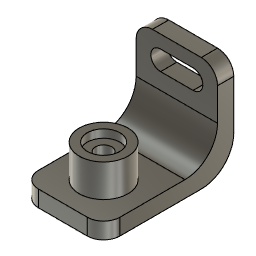
Tarea09_Ej1_jaalobuela (Autodesk Fusion 360 design; units mm, degrees)
Autodesk Fusion 360 part; units mm, degrees
sketch "Sketch1" plane through (0, 0, 0) normal (0, 0, 1) x (1, 0, 0)
  line L0 (-50, 25) -> (-41.3397, 30)
  line L1 (-50, 25) -> (-50, 35)
  line L2 (-50, 25) -> (-58.6603, 30)
  line L3 (-41.3397, 30) -> (-41.3397, 40)
  line L4 (-58.6603, 30) -> (-58.6603, 40)
  line L5 (-50, 35) -> (-41.3397, 40)
  line L6 (-50, 35) -> (-58.6603, 40)
  line L7 (-50, 45) -> (-41.3397, 40)
  line L8 (-50, 45) -> (-58.6603, 40)
sketch "Sketch2" plane through (0, 0, 0) normal (0, 0, 1) x (1, 0, 0)
  line L0 (-52.3894, 55.4322) -> (-22.3894, 55.4322)
  line L1 (-12.3894, 45.4322) -> (-12.3894, 15.4322)
  line L2 (-22.3894, 5.4322) -> (-52.3894, 5.4322)
  line L3 (-62.3894, 15.4322) -> (-62.3894, 45.4322)
  arc A0 (-12.3894, 45.4322) -> (-22.3894, 55.4322) centre (-22.3894, 45.4322) ccw
  arc A1 (-22.3894, 5.4322) -> (-12.3894, 15.4322) centre (-22.3894, 15.4322) ccw
  circle A2 through (-32.3894, 30.4322, 10) (-39.8894, 34.7623, 10) (-39.8894, 26.102, 10)
  circle A3 through (-27.3894, 30.4322, 10) (-42.3894, 39.0924, 10) (-42.3894, 21.7719, 10)
  circle A4 through (-22.3894, 30.4322, 10) (-44.8894, 43.4225, 10) (-44.8894, 17.4418, 10)
  line L4 (-37.3894, 55.4322) -> (-37.3894, 5.4322) construction
  line L5 (-62.3894, 30.4322) -> (-12.3894, 30.4322)
  line L6 (-62.3894, 15.4322) -> (-62.3894, 5.4322)
  line L7 (-62.3894, 45.4322) -> (-62.3894, 55.4322)
  line L8 (-52.3894, 55.4322) -> (-62.3894, 55.4322)
  line L9 (-52.3894, 5.4322) -> (-62.3894, 5.4322)
  point P0 (-12.3894, 55.4322)
  dimension "d8" = 50
  dimension "d9" = 50
  constraint horizontal L0
  constraint vertical L1
  constraint horizontal L2
  constraint vertical L3
  constraint coincident L7.end L0
  constraint coincident L7.end L3
  constraint coincident L6.end L3
  constraint coincident L6.end L2
  constraint coincident P0 L0
  constraint coincident P0 L1
  constraint tangent L0 A0
  constraint tangent L1 A0
  constraint tangent L1 A1
  constraint tangent L2 A1
  constraint midpoint L0 L4.start
  constraint midpoint L2 L4.end
  constraint midpoint L3 L5.start
  constraint midpoint L1 L5.end
  constraint parallel L3 L6
  constraint parallel L3 L7
  constraint perpendicular L7 L8
  constraint perpendicular L3 L9
  measures "d8" distance of L7.end P0
  measures "d9" distance of L7.end L6.end
extrude "Extrude1" add sketch "Sketch2" along normal blind 10 makes body 1
extrude "Extrude2" add sketch "Sketch2" along normal blind 15 contours A3 in plane through (0, 0, 10) normal (0, 0, 1) bodies 1
extrude "Extrude3" add sketch "Sketch2" along normal blind 20 contours A4 in plane through (0, 0, 10) normal (0, 0, 1) bodies 1
sketch "Sketch3" plane through (0, 0, 0) normal (1, 0, 0) x (0, 1, 0)
  line L0 (13, 99) -> (43, 99)
  line L1 (53, 89) -> (53, 49)
  line L2 (53, 49) -> (3, 49)
  line L3 (3, 49) -> (3, 89)
  arc A0 (13, 99) -> (3, 89) centre (13, 89) ccw
  arc A1 (53, 89) -> (43, 99) centre (43, 89) ccw
  line L4 (28, 99) -> (28, 91) construction
  line L5 (28, 91) -> (38, 91)
  line L6 (38, 79) -> (28, 79)
  line L7 (28, 91) -> (18, 91)
  line L8 (18, 79) -> (28, 79)
  arc A2 (18, 91) -> (18, 79) centre (18, 85) ccw
  arc A3 (38, 79) -> (38, 91) centre (38, 85) ccw
  point P0 (3, 99)
  point P1 (53, 99)
  dimension "d21" = 50
  dimension "d22" = 50
  dimension "d23" = 10
  dimension "d24" = 10
  dimension "d25" = 8
  dimension "d27" = 10
  constraint horizontal L0
  constraint vertical L1
  constraint horizontal L2
  constraint vertical L3
  constraint coincident P0 L0
  constraint coincident P0 L3
  constraint tangent L0 A0
  constraint tangent L3 A0
  constraint coincident P1 L0
  constraint coincident P1 L1
  constraint tangent L0 A1
  constraint tangent L1 A1
  constraint midpoint L0 L4.start
  constraint perpendicular L0 L4
  measures "d21" distance of P0 P1
  measures "d22" distance of P0 L2.end
  measures "d23" radius of A0
  measures "d24" radius of A1
  measures "d25" distance of L4.start L4.end
  measures "d27" distance of L4.end L5.end
extrude "Extrude4" add sketch "Sketch3" along normal blind 10 separate body makes body 2
move_face "OffsetFaces1" offset 20 1 faces at (-62.3894, 22.0988, 3.3333) on bodies 1
extrude "Extrude5" add 1 faces at (3.3333, 36.3333, 49) along direction (0, 0, -1) blind 10 on bodies 2 bodies 2
move_body "Move1" bodies 2 to x (1, 0, 0) y (0, 1, 0) z (0, 0, 1) at (-92.3894, 2.4322, -39)
combine "Combine1" operation add target body 1 tool bodies 2
fillet "Fillet1" radius 20 1 edges at (-82.3894, 30.4322, 10) on bodies 1
fillet "Fillet2" radius 20 1 edges at (-92.3894, 30.4322, 0) on bodies 1
move_body "Move2" bodies 1 to x (0, -1, 0) y (1, 0, 0) z (0, 0, 1) at (-67.8216, -6.9573, 0)
